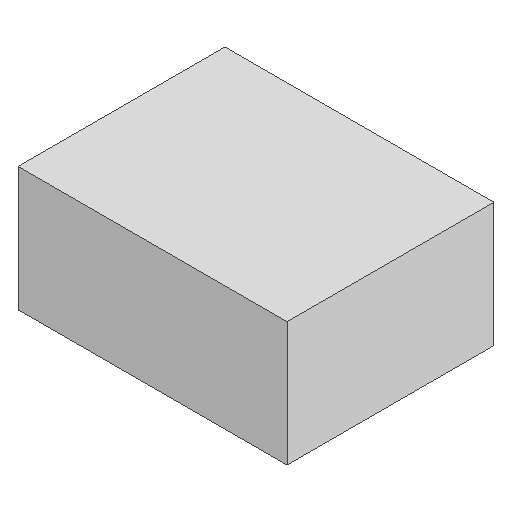
# Autodesk Inventor part: USB_A
Saved by Autodesk Inventor 2025.2 (Build 292293000, 293)
## iProperties
Created: 2025-03-09
Part Number: USB_A
Material: Generic
Document SubType Name: Modeling
Designer: ahorat
Density: 1 g/cm^3
Appearance: Default
Author: ahorat
Autodesk Inventor part; units mm, degrees
ref_plane "YZ Plane" through (0, 0, 0) normal (1, 0, 0) x (0, 1, 0)
ref_plane "XZ Plane" through (0, 0, 0) normal (0, 1, 0) x (-1, 0, 0)
ref_plane "XY Plane" through (0, 0, 0) normal (0, 0, 1) x (1, 0, 0)
sketch "Sketch1" plane through (0, 0, 0) normal (0, 0, 1) x (1, 0, 0)
  line L0 (-6.5, 6) -> (6.5, 6)
  line L1 (6.5, 6) -> (6.5, 0)
  line L2 (6.5, 0) -> (-6.5, 0)
  line L3 (-6.5, 0) -> (-6.5, 6)
  point P0 (0, 0)
  point P1 (0, 0)
  dimension "d0" = 13
  dimension "d1" = 6
  constraints: 8 end point, 2 parallel, 1 coincident, 1 horizontal, 1 midpoint, 1 perpendicular
  measures "d0" distance of L0.start L0.end
  measures "d1" distance of L0.end L1.end
extrude "Extrusion1" add sketch "Sketch1" along normal blind 10
sketch "Sketch2" plane through (-6.5, 0, 0) normal (0, 0, -1) x (-1, 0, 0)
  line L0 (-0.2, 5.8) -> (-12.8, 5.8)
  line L1 (-12.8, 5.8) -> (-12.8, 0.2)
  line L2 (-12.8, 0.2) -> (-0.2, 0.2)
  line L3 (-0.2, 0.2) -> (-0.2, 5.8)
  line L4 (-12.25, 4.8) -> (-0.75, 4.8)
  line L5 (-0.75, 4.8) -> (-0.75, 3)
  line L6 (-0.75, 3) -> (-12.25, 3)
  line L7 (-12.25, 3) -> (-12.25, 4.8)
  line L8 (0, 6) -> (0, 0) projected
  line L9 (0, 0) -> (-13, 0) projected
  line L10 (-13, 6) -> (0, 6) projected
  point P0 (-6.5, 0)
  point P1 (-12.8, 3)
  point P2 (-6.5, 5.8)
  point P3 (-6.5, 4.8)
  point P4 (-0.2, 3)
  point P5 (0, 3)
  point P6 (-6.5, 0)
  point P7 (-6.5, 0)
  dimension "d4" = 11.5
  dimension "d5" = 0.2
  dimension "d6" = 0.2
  dimension "d7" = 3
  dimension "d8" = 1
  constraints: 16 end point, 7 midpoint, 4 parallel, 3 vertical alignment, 2 horizontal, 2 perpendicular, 1 coincident, 1 horizontal alignment
  measures "d4" distance of L4.start L4.end
  measures "d5" distance between parallel lines of L10 L0
  measures "d6" distance between parallel lines of L8 L3
  measures "d7" distance between parallel lines of L10 L6
  measures "d8" distance between parallel lines of L0 L4
extrude "Extrusion2" cut sketch "Sketch2" against normal blind 9.8
body "Solid1"
